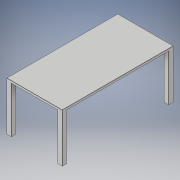
# Autodesk Inventor part: Table
Saved by Autodesk Inventor 2018 (Build 220112000, 112)
## iProperties
Created: 2019-10-17
Part Number: Table
Material: Generic
Document SubType Name: Modeling
Designer: Jacob
Density: 1 g/cm^3
Appearance: Default
Author: Jacob
Autodesk Inventor part; units mm, degrees
ref_plane "YZ Plane" through (0, 0, 0) normal (1, 0, 0) x (0, 1, 0)
ref_plane "XZ Plane" through (0, 0, 0) normal (0, 1, 0) x (-1, 0, 0)
ref_plane "XY Plane" through (0, 0, 0) normal (0, 0, 1) x (1, 0, 0)
sketch "Sketch1" plane through (0, 0, 0) normal (0, 1, 0) x (-1, 0, 0)
  line L0 (457.2, 914.4) -> (-457.2, 914.4)
  line L1 (-457.2, 914.4) -> (-457.2, -914.4)
  line L2 (-457.2, -914.4) -> (457.2, -914.4)
  line L3 (457.2, -914.4) -> (457.2, 914.4)
  line L4 (457.2, 914.4) -> (-457.2, -914.4) construction
  line L5 (-457.2, 914.4) -> (457.2, -914.4) construction
  point P0 (0, 0)
  dimension "d0" = 1828.8
  dimension "d1" = 914.4
  constraints: 12 end point, 2 midpoint, 2 parallel, 1 horizontal, 1 perpendicular
  measures "d0" distance of L2.end L0.start
  measures "d1" distance of L1.end L2.end
extrude "Extrusion1" add sketch "Sketch1" along normal blind 38.1
sketch "Sketch2" plane through (0, 0, 0) normal (0, -1, 0) x (1, 0, 0)
  line L0 (-457.2, 914.4) -> (457.2, 914.4) projected
  line L1 (457.2, 914.4) -> (381, 914.4)
  line L2 (381, 914.4) -> (381, 838.2)
  line L3 (381, 838.2) -> (457.2, 838.2)
  line L4 (457.2, 838.2) -> (457.2, 914.4)
  line L5 (-457.2, -914.4) -> (-457.2, 914.4) projected
  line L6 (-457.2, 914.4) -> (-381, 914.4)
  line L7 (-381, 914.4) -> (-381, 838.2)
  line L8 (-381, 838.2) -> (-457.2, 838.2)
  line L9 (-457.2, 838.2) -> (-457.2, 914.4)
  line L10 (-457.2, -914.4) -> (-381, -914.4)
  line L11 (-381, -914.4) -> (-381, -838.2)
  line L12 (-381, -838.2) -> (-457.2, -838.2)
  line L13 (-457.2, -838.2) -> (-457.2, -914.4)
  line L14 (457.2, 914.4) -> (457.2, -914.4) projected
  line L15 (457.2, -914.4) -> (381, -914.4)
  line L16 (381, -914.4) -> (381, -838.2)
  line L17 (381, -838.2) -> (457.2, -838.2)
  line L18 (457.2, -838.2) -> (457.2, -914.4)
  point P0 (0, 0)
  dimension "d4" = 76.2
  dimension "d5" = 76.2
  dimension "d6" = 76.2
  dimension "d7" = 76.2
  dimension "d8" = 76.2
  dimension "d9" = 76.2
  dimension "d10" = 76.2
  dimension "d11" = 76.2
  constraints: 32 end point, 8 parallel, 4 horizontal, 4 perpendicular
  measures "d4" distance of L16.end L17.end
  measures "d5" distance of L15.end L16.end
  measures "d6" distance of L10.end L11.end
  measures "d7" distance of L11.end L12.end
  measures "d8" distance of L6.end L7.end
  measures "d9" distance of L7.end L8.end
  measures "d10" distance of L1.end L2.end
  measures "d11" distance of L2.end L3.end
extrude "Extrusion2" add sketch "Sketch2" along normal blind 762
fillet "Fillet1" radius 3.175 23 edges at (457.2, 38.1, 0) (0, 38.1, -914.4) (-457.2, 38.1, 0) (0, 38.1, 914.4) (457.2, 0, 0) (0, 0, -914.4) (-457.2, 0, 0) (0, 0, 914.4) (-457.2, -361.95, 914.4) (-381, -381, 914.4) (-457.2, -381, 838.2) (381, -381, 914.4) (381, -381, 838.2) (457.2, -361.95, 914.4) (-381, -381, -838.2) (-457.2, -381, -838.2) (-457.2, -361.95, -914.4) (-381, -381, 838.2) (457.2, -381, 838.2) (381, -381, -838.2) (457.2, -381, -838.2) (457.2, -361.95, -914.4) (381, -381, -914.4)
body "Solid1"
